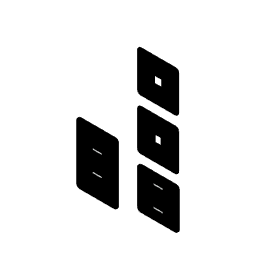
Acrylic Plates & Foam v3 (Autodesk Fusion 360 design; units mm, degrees)
Autodesk Fusion 360 part; units mm, degrees
sketch "Sketch1" plane through (0, 0, 0) normal (0, 1, 0) x (1, 0, 0)
  line L0 (100, -100) -> (-100, -100)
  line L1 (-100, -100) -> (-100, 100)
  line L2 (-100, 100) -> (100, 100)
  line L3 (100, 100) -> (100, -100)
  line L4 (100, -100) -> (-100, 100) construction
  line L5 (-100, -100) -> (100, 100) construction
  dimension "d1" = 200
  dimension "d2" = 200
  constraint horizontal L0
  constraint perpendicular L0 L1
  constraint parallel L0 L2
  constraint parallel L1 L3
  constraint coincident L4 origin
  constraint coincident L5 origin
  measures "d1" distance of L1.end L2.end
  measures "d2" distance of L0.end L1.end
extrude "Extrude1" add sketch "Sketch1" along normal blind 3 makes body 1
fillet "Fillet1" radius 15 4 edges at (100, 1.5, 100) (-100, 1.5, 100) (100, 1.5, -100) (-100, 1.5, -100) on bodies 1
sketch "Sketch2" plane through (0, 0, 0) normal (0, -1, 0) x (1, 0, 0)
  arc A0 (-100, -85) -> (-85, -100) centre (-85, -85) ccw
  line L0 (-85, -100) -> (85, -100)
  arc A1 (85, -100) -> (100, -85) centre (85, -85) ccw
  line L1 (100, -85) -> (100, 85)
  arc A2 (100, 85) -> (85, 100) centre (85, 85) ccw
  line L2 (85, 100) -> (-85, 100)
  arc A3 (-85, 100) -> (-100, 85) centre (-85, 85) ccw
  line L3 (-100, 85) -> (-100, -85)
  line L4 (0, 0) -> (0, 50) construction
  line L5 (25.5, 56.5) -> (-25.5, 56.5)
  line L6 (-25.5, 56.5) -> (-25.5, 43.5)
  line L7 (-25.5, 43.5) -> (25.5, 43.5)
  line L8 (25.5, 43.5) -> (25.5, 56.5)
  line L9 (25.5, 56.5) -> (-25.5, 43.5) construction
  line L10 (-25.5, 56.5) -> (25.5, 43.5) construction
  line L11 (0, 0) -> (29, 0) construction
  line L12 (-25.5, -56.5) -> (25.5, -43.5) construction
  line L13 (25.5, -56.5) -> (-25.5, -56.5)
  line L14 (-25.5, -43.5) -> (25.5, -43.5)
  line L15 (25.5, -56.5) -> (-25.5, -43.5) construction
  line L16 (-25.5, -56.5) -> (-25.5, -43.5)
  line L17 (25.5, -43.5) -> (25.5, -56.5)
  point P0 (0, 50)
  point P1 (0, -50)
  point P2 (0, -50)
  dimension "d7" = 50
  dimension "d9" = 51
  dimension "d10" = 13
  constraint vertical L4
  constraint coincident L4.start L11.start
  constraint horizontal L5
  constraint perpendicular L5 L6
  constraint parallel L5 L7
  constraint parallel L6 L8
  constraint coincident L9 P0
  constraint coincident L10 P0
  constraint coincident P0 L4.end
  constraint perpendicular L4 L11
  constraint symmetric P0 L11 P2
  constraint symmetric L5.start L11 L13.start
  constraint symmetric L5.end L11 L12.start
  constraint symmetric L6.end L11 L14.start
  constraint symmetric L7.end L11 L12.end
  measures "d7" distance of L4.start P0
  measures "d9" distance of L6.end L7.end
  measures "d10" distance of L5.end L6.end
extrude "Extrude1'" add sketch "Sketch2" along normal blind 2 separate body makes body 2 in component "Foam Protector"
copy_body "Body->Comp1" bodies 1 removing the originals makes body 3 in component "Acrylic sheet"
sketch "Sketch1 (2)" plane through (0, 0, 0) normal (0, 1, 0) x (1, 0, 0) in component "Acrylic sheet"
  line L0 (100, -150) -> (-100, -150)
  line L1 (-100, -150) -> (-100, 150)
  line L2 (-100, 150) -> (100, 150)
  line L3 (100, 150) -> (100, -150)
  line L4 (100, -150) -> (-100, 150) construction
  line L5 (-100, -150) -> (100, 150) construction
  dimension "d15" = 200
  dimension "d16" = 300
  constraint horizontal L0
  constraint perpendicular L0 L1
  constraint parallel L0 L2
  constraint parallel L1 L3
  constraint coincident L4 origin
  constraint coincident L5 origin
  measures "d15" distance of L1.end L2.end
  measures "d16" distance of L0.end L1.end
extrude "Extrude1''" add sketch "Sketch1 (2)" along normal blind 3 separate body makes body 4 in component "Acrylic sheet"
fillet "Fillet1'" radius 15 4 edges at (100, 1.5, 150) (-100, 1.5, 150) (100, 1.5, -150) (-100, 1.5, -150) on bodies 4 in component "Acrylic sheet"
sketch "Sketch1 (3)" plane through (0, 0, 0) normal (0, -1, 0) x (1, 0, 0) in component "Foam Protector"
  arc A0 (-100, -135) -> (-85, -150) centre (-85, -135) ccw
  line L0 (-85, -150) -> (85, -150)
  arc A1 (85, -150) -> (100, -135) centre (85, -135) ccw
  line L1 (100, -135) -> (100, 135)
  arc A2 (100, 135) -> (85, 150) centre (85, 135) ccw
  line L2 (85, 150) -> (-85, 150)
  arc A3 (-85, 150) -> (-100, 135) centre (-85, 135) ccw
  line L3 (-100, 135) -> (-100, -135)
  line L4 (0, 0) -> (0, 50) construction
  line L5 (0, 0) -> (15, 0) construction
  line L6 (25.5, 56.5) -> (-25.5, 56.5)
  line L7 (-25.5, 56.5) -> (-25.5, 43.5)
  line L8 (-25.5, 43.5) -> (25.5, 43.5)
  line L9 (25.5, 43.5) -> (25.5, 56.5)
  line L10 (25.5, 56.5) -> (-25.5, 43.5) construction
  line L11 (-25.5, 56.5) -> (25.5, 43.5) construction
  line L12 (-25.5, -56.5) -> (25.5, -43.5) construction
  line L13 (25.5, -56.5) -> (-25.5, -43.5) construction
  line L14 (25.5, -43.5) -> (25.5, -56.5)
  line L15 (-25.5, -56.5) -> (-25.5, -43.5)
  line L16 (-25.5, -43.5) -> (25.5, -43.5)
  line L17 (25.5, -56.5) -> (-25.5, -56.5)
  point P0 (0, 50)
  point P1 (0, -50)
  point P2 (0, -50)
  dimension "d21" = 50
  dimension "d22" = 51
  dimension "d23" = 13
  constraint vertical L4
  constraint coincident L4.start L5.start
  constraint perpendicular L4 L5
  constraint horizontal L6
  constraint perpendicular L6 L7
  constraint parallel L6 L8
  constraint parallel L7 L9
  constraint coincident L10 P0
  constraint coincident L11 P0
  constraint coincident P0 L4.end
  constraint symmetric P0 L5 P2
  constraint symmetric L5 L6.start L13.start
  constraint symmetric L5 L6.end L12.start
  constraint symmetric L5 L7.end L13.end
  constraint symmetric L5 L8.end L12.end
  constraint symmetric L5 P0 P2
  measures "d21" distance of L4.start P0
  measures "d22" distance of L7.end L8.end
  measures "d23" distance of L6.end L7.end
extrude "Extrude2" add sketch "Sketch1 (3)" along normal blind 2 separate body makes body 5 in component "Foam Protector"
fillet "Fillet1''" radius 2.5 4 edges at (-25.5, -1, 43.5) (-25.5, -1, 56.5) (25.5, -1, 43.5) (25.5, -1, 56.5) on bodies 5 in component "Foam Protector"
fillet "Fillet1''" radius 2.5 4 edges at (25.5, -1, -43.5) (25.5, -1, -56.5) (-25.5, -1, -43.5) (-25.5, -1, -56.5) on bodies 5 in component "Foam Protector"
fillet "Fillet2" radius 2.5 4 edges at (-25.5, -1, -56.5) (-25.5, -1, -43.5) (25.5, -1, -56.5) (25.5, -1, -43.5) on bodies 2 in component "Foam Protector"
move_body "Move1" bodies 3 to x (1, 0, 0) y (0, 1, 0) z (0, 0, 1) at (300, 0, 0) in component "Acrylic sheet"
move_body "Move1'" bodies 2 to x (1, 0, 0) y (0, 1, 0) z (0, 0, 1) at (300, 0, 0) in component "Foam Protector"
sketch "Sketch2 (2)" plane through (0, 0, 0) normal (0, -1, 0) x (1, 0, 0) in component "Foam Protector"
  arc A0 (200, -85) -> (215, -100) centre (215, -85) ccw
  line L0 (215, -100) -> (385, -100)
  arc A1 (385, -100) -> (400, -85) centre (385, -85) ccw
  line L1 (400, -85) -> (400, 85)
  arc A2 (400, 85) -> (385, 100) centre (385, 85) ccw
  line L2 (385, 100) -> (215, 100)
  arc A3 (215, 100) -> (200, 85) centre (215, 85) ccw
  line L3 (200, 85) -> (200, -85)
  line L4 (300, 100) -> (300, 0) construction
  line L5 (315.5, 18.5) -> (284.5, 18.5)
  line L6 (284.5, 18.5) -> (284.5, -18.5)
  line L7 (284.5, -18.5) -> (315.5, -18.5)
  line L8 (315.5, -18.5) -> (315.5, 18.5)
  line L9 (315.5, 18.5) -> (284.5, -18.5) construction
  line L10 (284.5, 18.5) -> (315.5, -18.5) construction
  point P0 (300, 0)
  dimension "d32" = 31
  dimension "d33" = 37
  constraint midpoint L2 L4.start
  constraint perpendicular L2 L4
  constraint horizontal L5
  constraint perpendicular L5 L6
  constraint parallel L5 L7
  constraint parallel L6 L8
  constraint coincident L9 P0
  constraint coincident L10 P0
  constraint coincident P0 L4.end
  measures "d32" distance of L6.end L7.end
  measures "d33" distance of L5.end L6.end
extrude "Extrude3" add sketch "Sketch2 (2)" along normal blind 2 separate body makes body 6 in component "Foam Protector"
sketch "Sketch3" plane through (0, 0, 0) normal (0, -1, 0) x (1, 0, 0) in component "Foam Protector"
  arc A0 (200, -85) -> (215, -100) centre (215, -85) ccw
  line L0 (215, -100) -> (385, -100)
  arc A1 (385, -100) -> (400, -85) centre (385, -85) ccw
  line L1 (400, -85) -> (400, 85)
  arc A2 (400, 85) -> (385, 100) centre (385, 85) ccw
  line L2 (385, 100) -> (215, 100)
  arc A3 (215, 100) -> (200, 85) centre (215, 85) ccw
  line L3 (200, 85) -> (200, -85)
  line L4 (300, 100) -> (300, 0) construction
  line L5 (318.75, 18.5) -> (281.25, 18.5)
  line L6 (281.25, 18.5) -> (281.25, -18.5)
  line L7 (281.25, -18.5) -> (318.75, -18.5)
  line L8 (318.75, -18.5) -> (318.75, 18.5)
  line L9 (318.75, 18.5) -> (281.25, -18.5) construction
  line L10 (281.25, 18.5) -> (318.75, -18.5) construction
  point P0 (300, 0)
  dimension "d36" = 100
  dimension "d37" = 37.5
  dimension "d38" = 37
  constraint vertical L4
  constraint midpoint L2 L4.start
  constraint horizontal L5
  constraint perpendicular L5 L6
  constraint parallel L5 L7
  constraint parallel L6 L8
  constraint coincident L9 P0
  constraint coincident L10 P0
  constraint coincident P0 L4.end
  measures "d36" distance of L4.start P0
  measures "d37" distance of L6.end L7.end
  measures "d38" distance of L5.end L6.end
extrude "Extrude4" add sketch "Sketch3" along normal blind 2 separate body makes body 7 in component "Foam Protector"
move_body "Move2" bodies 6 to x (1, 0, 0) y (0, 1, 0) z (0, 0, 1) at (0, 0, 250) in component "Foam Protector"
move_body "Move3" bodies 7 to x (1, 0, 0) y (0, 1, 0) z (0, 0, 1) at (0, 0, 500) in component "Foam Protector"
component "Foam Protector" placed x (1, 0, 0) y (0, 1, 0) z (0, 0, 1) at (0, 0, 0)
component "Acrylic sheet" placed x (1, 0, 0) y (0, 1, 0) z (0, 0, 1) at (0, 0, 0)
equation "d32 = 30 mm + 1 mm"
equation "d33 = ( 12 * 3 ) * 1 mm + 1 mm"
equation "d37 = 36.5 mm + 1 mm"
equation "d38 = ( 12 * 3 ) * 1 mm + 1 mm"
named bodies: "200x200 - Double 1x7", "200x200", "200x300", "200x300 - Double 1x7", "200x200 - Single 3x4", "200x200-Single 3x5"
